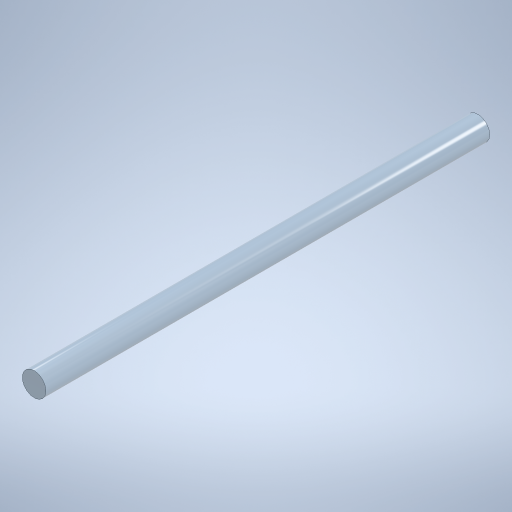
# Autodesk Inventor part: ACME Lead Screw 8mm
Saved by Autodesk Inventor 2023.1 (Build 271208000, 208)
## iProperties
Created: 2023-01-19
Part Number: ACME Lead Screw 8mm
Material: Stainless Steel
Document SubType Name: Modeling
Designer: dmargari
Density: 8 g/cm^3
Appearance: Steel Blue
Author: dmargari
Autodesk Inventor part; units mm, degrees
ref_plane "YZ Plane" through (0, 0, 0) normal (1, 0, 0) x (0, 1, 0)
ref_plane "XZ Plane" through (0, 0, 0) normal (0, 1, 0) x (-1, 0, 0)
ref_plane "XY Plane" through (0, 0, 0) normal (0, 0, 1) x (1, 0, 0)
sketch "Sketch1" plane through (0, 0, 0) normal (0, 0, 1) x (1, 0, 0)
  circle A0 centre (10.5742, 11.4503) radius 4
  point P0 (0, 0)
  dimension "d0" = 8
  dimension "d0" = 8
  constraints: 1 centre point
  measures "d0" diameter of A0
extrude "Extrusion1" add sketch "Sketch1" along normal mid plane 150
body "Solid1"
